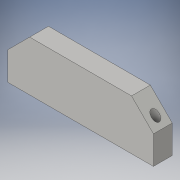
# Autodesk Inventor part: Voltage Divider (Rough)
Saved by Autodesk Inventor 2016 (Build 200138000, 138)
## iProperties
Created: 2017-10-13
Part Number: Voltage Divider (Rough)
Material: Generic
Document SubType Name: Modeling
Designer: Student
Density: 1 g/cm^3
Appearance: Default
Author: Student
Autodesk Inventor part; units mm, degrees
ref_plane "YZ Plane" through (0, 0, 0) normal (1, 0, 0) x (0, 1, 0)
ref_plane "XZ Plane" through (0, 0, 0) normal (0, 1, 0) x (-1, 0, 0)
ref_plane "XY Plane" through (0, 0, 0) normal (0, 0, 1) x (1, 0, 0)
sketch "Sketch1" plane through (0, 0, 0) normal (0, 1, 0) x (-1, 0, 0)
  line L0 (-39.2837, 182.0907) -> (45.1561, 182.0907)
  line L1 (45.1561, 182.0907) -> (45.1561, 192.9873)
  line L2 (-39.2837, 192.9873) -> (-39.2837, 182.0907)
  circle A0 centre (40.7951, 187.539) radius 2.2274
  circle A1 centre (-34.9227, 187.539) radius 2.2274
  line L3 (52.1157, -152.8547) -> (52.1157, 254.4851) construction
  line L4 (-39.2837, 182.0907) -> (45.1561, 182.0907) construction
  line L5 (45.1561, 182.0907) -> (45.1561, 192.9873) construction
  line L6 (45.1561, 192.9873) -> (-39.2837, 192.9873)
  line L7 (-39.2837, 192.9873) -> (-39.2837, 182.0907) construction
  circle A2 centre (40.7951, 187.539) radius 2.2274
  circle A3 centre (-34.9227, 187.539) radius 2.2274
  line L8 (-47.9603, 254.4851) -> (-47.9603, -152.8547) construction
  line L9 (45.1561, 166.5182) -> (-39.2837, 166.5182)
  line L10 (-39.2837, 166.5182) -> (-39.2837, 155.6216)
  line L11 (-39.2837, 155.6216) -> (45.1561, 155.6216)
  line L12 (45.1561, 155.6216) -> (45.1561, 166.5182)
  circle A4 centre (40.7951, 161.0699) radius 2.2274
  circle A5 centre (-34.9227, 161.0699) radius 2.2274
  point P0 (0, 0)
  point P1 (0, 0)
  point P2 (0, 0)
  dimension "d0" = 84.4398
  dimension "d1" = 10.8966
  dimension "d3" = 2.1336
  dimension "d4" = 2.1336
  dimension "d5" = 6.9596
  dimension "d6" = 84.4398
  dimension "d7" = 10.8966
  dimension "d9" = 2.1336
  dimension "d10" = 2.1336
  dimension "d14" = 10.8966
  dimension "d15" = 3.2209
  dimension "d16" = 3.2209
  dimension "d17" = 2.1336
  dimension "d18" = 2.1336
  dimension "d19" = 3.2209
  dimension "d20" = 3.2209
  dimension "d21" = 75.7178
  dimension "d22" = 75.7178
  dimension "d23" = 84.4398
  constraints: 26 end point, 7 perpendicular, 6 centre point, 3 horizontal
  measures "d0" distance of L1.end L2.start
  measures "d1" distance of L2.start L0.start
  measures "d3" distance edge to line of A0 L1
  measures "d4" distance edge to line of A1 L2
  measures "d5" distance between parallel lines of L3 L1
  measures "d6" distance of L5.end L6.end
  measures "d7" distance of L6.end L4.start
  measures "d9" distance edge to line of A2 L5
  measures "d10" distance edge to line of A3 L7
  measures "d14" distance of L11.end L9.start
  measures "d15" distance edge to line of A0 L0
  measures "d16" distance edge to line of A1 L0
  measures "d17" distance edge to line of A4 L12
  measures "d18" distance edge to line of A5 L10
  measures "d19" distance edge to line of A4 L11
  measures "d20" distance edge to line of A5 L11
  measures "d21" distance of A1.centre A0.centre
  measures "d22" distance of A5.centre A4.centre
  measures "d23" distance of L9.start L9.end
extrude "Extrusion1" add sketch "Sketch1" along normal blind 29.0322 contours L12 L11 L10 L9
chamfer "Chamfer1" distance 12.7 angle 45 2 edges at (39.2837, 29.0322, 161.0699) (-45.1561, 29.0322, 161.0699)
equation "\"d4\" = d3"
equation "\"d10\" = d9"
equation "\"d14\" = d7"
equation "\"d17\" = d9"
equation "\"d18\" = d10"
equation "\"d19\" = d15"
equation "\"d20\" = d16"
body "Solid1"
